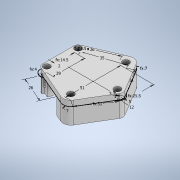
# Autodesk Inventor part: shaft adapter 2
Saved by Autodesk Inventor 2020.3 (Build 243373000, 373)
## iProperties
Created: 2020-09-11
Part Number: shaft adapter 2
Material: Generic
Document SubType Name: Modeling
Designer: joesp
Density: 1 g/cm^3
Appearance: Default
Author: joesp
Autodesk Inventor part; units mm, degrees
ref_plane "YZ Plane" through (0, 0, 0) normal (1, 0, 0) x (0, 1, 0)
ref_plane "XZ Plane" through (0, 0, 0) normal (0, 1, 0) x (-1, 0, 0)
ref_plane "XY Plane" through (0, 0, 0) normal (0, 0, 1) x (1, 0, 0)
sketch "Sketch1" plane through (0, 0, 0) normal (0, 1, 0) x (-1, 0, 0)
  circle A0 centre (50.8546, 14.5) radius 1.5
  circle A1 centre (50.8546, -14.5) radius 1.5
  circle A2 centre (17.6281, 25.5) radius 1.5
  circle A3 centre (0, 0) radius 1.5
  circle A4 centre (17.6281, -25.5) radius 1.5
  circle A5 centre (0, 0) radius 6
  circle A6 centre (17.6281, -25.5) radius 6
  circle A7 centre (50.8546, -14.5) radius 6
  circle A8 centre (50.8546, 14.5) radius 6
  circle A9 centre (17.6281, 25.5) radius 6
  arc A10 (-4.2878, 2.572) -> (-4.2878, -2.572) centre (0, 0) ccw
  arc A11 (20.3896, 31.9323) -> (11.6252, 29.1008) centre (17.6281, 25.5) ccw
  arc A12 (54.8546, 14.5) -> (52.4326, 18.1756) centre (50.8546, 14.5) ccw
  arc A13 (52.4326, -18.1756) -> (54.8546, -14.5) centre (50.8546, -14.5) ccw
  arc A14 (11.6252, -29.1008) -> (20.3896, -31.9323) centre (17.6281, -25.5) ccw
  line L0 (11.6252, 29.1008) -> (-4.2878, 2.572)
  line L1 (20.3896, 31.9323) -> (52.4326, 18.1756)
  line L2 (54.8546, 14.5) -> (54.8546, -14.5)
  line L3 (52.4326, -18.1756) -> (20.3896, -31.9323)
  line L4 (11.6252, -29.1008) -> (-4.2878, -2.572)
  line L5 (19.6006, 30.0945) -> (51.6436, 16.3378)
  arc A15 (52.8546, 14.5) -> (51.6436, 16.3378) centre (50.8546, 14.5) ccw
  arc A16 (51.6436, -16.3378) -> (52.8546, -14.5) centre (50.8546, -14.5) ccw
  arc A17 (13.3403, -28.072) -> (19.6006, -30.0945) centre (17.6281, -25.5) ccw
  arc A18 (-2.5727, 1.5432) -> (-2.5727, -1.5432) centre (0, 0) ccw
  arc A19 (19.6006, 30.0945) -> (13.3403, 28.072) centre (17.6281, 25.5) ccw
  line L6 (13.3403, 28.072) -> (-2.5727, 1.5432)
  line L7 (-2.5727, -1.5432) -> (13.3403, -28.072)
  line L8 (19.6006, -30.0945) -> (51.6436, -16.3378)
  line L9 (52.8546, -14.5) -> (52.8546, 14.5)
  line L10 (27.163, 29.0243) -> (26.374, 27.1865)
  line L11 (51.0543, 18.7673) -> (50.2653, 16.9295)
  line L12 (26.374, -27.1865) -> (27.163, -29.0243)
  line L13 (51.0543, -18.7673) -> (50.2653, -16.9295)
  point P0 (-6, 0)
  point P1 (48.3232, -19.9398)
  point P2 (54.8546, -10.0279)
  point P3 (54.8546, 10.0279)
  point P4 (48.3232, 19.9398)
  point P5 (50.9391, 18.4991)
  point P6 (46.4455, 18.5694)
  point P7 (52.8546, 8.8431)
  point P8 (52.8546, -8.8431)
  point P9 (46.4455, -18.5694)
  point P10 (50.9391, -18.4991)
  point P11 (0.1002, -5.9992)
  point P12 (0.1002, 5.9992)
  dimension "d0" = 51
  dimension "d1" = 25.5
  dimension "d2" = 31
  dimension "d3" = 31
  dimension "d4" = 29
  dimension "d5" = 14.5
  dimension "d6" = 35
  dimension "d7" = 3
  dimension "d8" = 12
  dimension "d9" = 6
  dimension "d23" = 7
  dimension "d24" = 7
  dimension "d25" = 5
  dimension "d26" = 4
  dimension "d27" = 4
  dimension "d30" = 2
  dimension "d31" = 26
  dimension "d32" = 1.5
  dimension "d33" = 26
  dimension "d34" = 1.5
  constraints: 28 end point, 20 centre point, 20 point on circle, 20 tangent, 17 coincident, 8 equal radius, 8 point on line, 4 perpendicular, 3 parallel, 2 vertical, 1 vertical alignment
  measures "d0" distance of A2.centre A4.centre
  measures "d1" vertical distance of A3.centre A4.centre
  measures "d2" distance of A3.centre A4.centre
  measures "d3" distance of A3.centre A2.centre
  measures "d4" distance of A0.centre A1.centre
  measures "d5" vertical distance of point (0, 0) A1.centre
  measures "d6" distance of A4.centre A1.centre
  measures "d7" diameter of A3
  measures "d8" diameter of A5
  measures "d9" distance of A5.centre point (-6, 0)
  measures "d23" radius of A11
  measures "d24" radius of A14
  measures "d25" radius of A10
  measures "d26" radius of A13
  measures "d27" radius of A12
  measures "d30" distance between parallel lines of L2 L9
  measures "d31" distance between parallel lines of L11 L10
  measures "d32" distance from line of L11 A0.centre
  measures "d33" distance between parallel lines of L13 L12
  measures "d34" distance from line of A1.centre L13
extrude "Extrusion1" add sketch "Sketch1" along normal blind 5 contours A5 L7 A18 L6 | A5 L6 A9 L5 A8 L9 A7 L8 A6 L7 | L6 A18 L7 A5 L4 A10 L0 | A5 L0 A11 L1 L10 L5 A9 L6 | L7 A6 L8 L12 L3 A14 L4 A5 | L6 A19 L5 A9 | A9 L5 A19 L6 | L7 A17 L8 A6 | A6 L8 A17 L7 | L10 L1 A8 L5 | L8 A7 L3 L12 | L5 A15 L9 A8 | A8 L1 L11 L5 | L8 L13 L3 A7 | A7 L9 A16 L8 | L9 A15 L5 L11 L1 A12 L2 A8 | A8 L2 A7 L9 | A7 L2 A13 L3 L13 L8 A16 L9
extrude "Extrusion2" add sketch "Sketch1" against normal blind 15 contours A5 L7 A18 L6 | L6 A18 L7 A5 L4 A10 L0 | A5 L0 A11 L1 L10 L5 A9 L6 | L7 A6 L8 L12 L3 A14 L4 A5 | L6 A19 L5 A9 | A9 L5 A19 L6 | L7 A17 L8 A6 | A6 L8 A17 L7 | L5 A15 L9 A8 | A7 L9 A16 L8 | L9 A15 L5 L11 L1 A12 L2 A8 | A8 L2 A7 L9 | A7 L2 A13 L3 L13 L8 A16 L9
sketch "Sketch2" plane through (0, 5, 0) normal (0, 1, 0) x (1, 0, 0)
  circle A0 centre (-50.8546, 14.5) radius 1.5 projected
  circle A1 centre (-50.8546, 14.5) radius 3
  circle A2 centre (-17.6281, 25.5) radius 3
  circle A3 centre (0, 0) radius 3
  circle A4 centre (-17.6281, -25.5) radius 3
  circle A5 centre (-50.8546, -14.5) radius 3
  circle A6 centre (-50.8546, -14.5) radius 1.5 projected
  circle A7 centre (-17.6281, -25.5) radius 1.5 projected
  circle A8 centre (-17.6281, 25.5) radius 1.5 projected
  circle A9 centre (0, 0) radius 1.5 projected
  dimension "d37" = 6
  constraints: 5 centre point, 4 concentric, 4 equal radius, 2 coincident
  measures "d37" diameter of A5
extrude "Extrusion3" cut sketch "Sketch2" against normal blind 15
equation "\"d1\" = 0.5 * d0"
equation "\"d3\" = d2"
equation "\"d5\" = 0.5 * d4"
body "Solid1"
